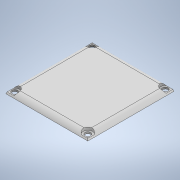
# Autodesk Inventor part: Lid-SensorHousing
Saved by Autodesk Inventor 2020 (Build 240168000, 168)
## iProperties
Created: 2022-06-20
Part Number: Lid-SensorHousing
Material: Generic
Document SubType Name: Modeling
Designer: Beaucage
Density: 1 g/cm^3
Appearance: Default
Author: Beaucage
Autodesk Inventor part; units mm, degrees
ref_plane "YZ Plane" through (0, 0, 0) normal (1, 0, 0) x (0, 1, 0)
ref_plane "XZ Plane" through (0, 0, 0) normal (0, 1, 0) x (-1, 0, 0)
ref_plane "XY Plane" through (0, 0, 0) normal (0, 0, 1) x (1, 0, 0)
sketch "Sketch1" plane through (0, 0, 0) normal (0, 1, 0) x (-1, 0, 0)
  line L0 (0, 0) -> (47.625, 0)
  line L1 (47.625, 0) -> (47.625, -50.165)
  line L2 (47.625, -50.165) -> (0, -50.165)
  line L3 (0, -50.165) -> (0, 0)
  dimension "d0" = 47.625
  dimension "d1" = 50.165
  constraints: 8 end point, 2 parallel, 1 horizontal, 1 perpendicular
  measures "d0" distance of L1.end L2.end
  measures "d1" distance of L0.end L1.end
extrude "Extrusion1" add sketch "Sketch1" along normal blind 2.54
sketch "Sketch2" plane through (0, 2.54, 0) normal (0, 1, 0) x (1, 0, 0)
  line L0 (-47.625, 0) -> (0, 0) projected
  line L1 (0, 0) -> (-2.54, 0)
  line L2 (-2.54, 0) -> (-2.54, 2.54)
  line L3 (-2.54, 2.54) -> (0, 2.54)
  line L4 (0, 2.54) -> (0, 0)
  line L5 (0, 0) -> (0, 50.165) projected
  line L6 (0, 50.165) -> (-2.54, 50.165)
  line L7 (-2.54, 50.165) -> (-2.54, 47.625)
  line L8 (-2.54, 47.625) -> (0, 47.625)
  line L9 (0, 47.625) -> (0, 50.165)
  line L10 (-47.625, 50.165) -> (-47.625, 0) projected
  line L11 (-47.625, 50.165) -> (-45.085, 50.165)
  line L12 (-45.085, 50.165) -> (-45.085, 47.625)
  line L13 (-45.085, 47.625) -> (-47.625, 47.625)
  line L14 (-47.625, 47.625) -> (-47.625, 50.165)
  line L15 (-47.625, 0) -> (-45.085, 0)
  line L16 (-45.085, 0) -> (-45.085, 2.54)
  line L17 (-45.085, 2.54) -> (-47.625, 2.54)
  line L18 (-47.625, 2.54) -> (-47.625, 0)
  dimension "d4" = 2.54
  dimension "d5" = 2.54
  dimension "d6" = 2.54
  dimension "d7" = 2.54
  constraints: 32 end point, 8 parallel, 6 point on line, 4 horizontal, 4 perpendicular
  measures "d4" distance of L2.end L3.end
  measures "d5" distance of L1.end L2.end
  measures "d6" distance of L7.end L6.end
  measures "d7" distance of L12.end L13.end
hole "Hole1" at (-45.085, 2.54, -47.625) at (-2.54, 2.54, -47.625) at (-2.54, 2.54, -2.54) at (-45.085, 2.54, -2.54) direction (0, -1, 0) diameter 3.2766 depth 7.2771 counterbore diameter 5.5626 counterbore depth 1.5875 clearance for "Socket Head Cap Screw" size "#4" standard "Ansi Unified Screw Threads"
fillet "Fillet1" radius 3.175 4 edges at (-23.8125, 2.54, 0) (0, 2.54, -25.0825) (-23.8125, 2.54, -50.165) (-47.625, 2.54, -25.0825)
body "Solid1"
